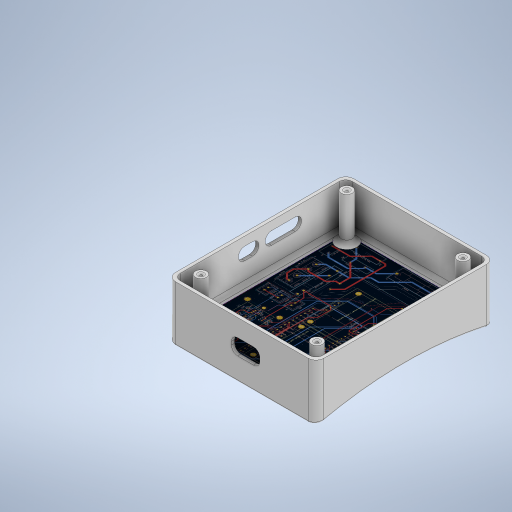
# Autodesk Inventor part: lautering_tank_box
Saved by Autodesk Inventor 2024.4 (Build 284460000, 460)
## iProperties
Created: 2026-05-24
Part Number: lautering_tank_box
Material: Generic
Document SubType Name: Modeling
Designer: Emil
Density: 1 g/cm^3
Appearance: Default
Author: Emil
Autodesk Inventor part; units mm, degrees
ref_plane "YZ Plane" through (0, 0, 0) normal (1, 0, 0) x (0, 1, 0)
ref_plane "XZ Plane" through (0, 0, 0) normal (0, 1, 0) x (-1, 0, 0)
ref_plane "XY Plane" through (0, 0, 0) normal (0, 0, 1) x (1, 0, 0)
sketch "Sketch1" plane through (0, 0, 0) normal (0, 1, 0) x (-1, 0, 0)
  line L0 (0, 0) -> (0, -100.838) construction
  line L1 (0, -100.838) -> (-82.0304, -100.838) construction
  line L2 (-82.0304, -100.838) -> (-82.0304, 0) construction
  line L3 (-82.0304, 0) -> (0, 0) construction
  point P0 (-41.0152, -50.419)
  point P1 (-41.0152, -50.419)
  constraints: 4 other
sketch "Sketch2" plane through (0, 0, 0) normal (0, 1, 0) x (-1, 0, 0)
  line L0 (-86.0304, 4) -> (4, 4)
  line L1 (4, 4) -> (4, -104.838)
  line L2 (4, -104.838) -> (-86.0304, -104.838)
  line L3 (-86.0304, -104.838) -> (-86.0304, 4)
  line L4 (-86.0304, 4) -> (4, -104.838) construction
  line L5 (4, 4) -> (-86.0304, -104.838) construction
  line L6 (-88.0304, 6) -> (6, 6)
  line L7 (6, 6) -> (6, -106.838)
  line L8 (6, -106.838) -> (-88.0304, -106.838)
  line L9 (-88.0304, -106.838) -> (-88.0304, 6)
  line L10 (-88.0304, 6) -> (6, -106.838) construction
  line L11 (6, 6) -> (-88.0304, -106.838) construction
  line L12 (0, -100.838) -> (-82.0304, -100.838) construction
  line L13 (-82.0304, 0) -> (0, 0) construction
  line L14 (0, 0) -> (0, -100.838) construction
  line L15 (-82.0304, -100.838) -> (-82.0304, 0) construction
  point P0 (-41.0152, -50.419)
  dimension "d28" = 4
  dimension "d29" = 2
  dimension "d30" = 4
  dimension "d31" = 2
  dimension "d96" = 94.0304
  dimension "d97" = 112.838
  constraints: 24 end point, 4 midpoint, 4 parallel, 2 horizontal, 2 perpendicular
  measures "d28" distance between parallel lines of L2 L12
  measures "d29" distance between parallel lines of L8 L2
  measures "d30" distance between parallel lines of L1 L14
  measures "d31" distance between parallel lines of L7 L1
  measures "d96" distance of L7.end L8.end
  measures "d97" distance of L8.end L6.start
extrude "Extrusion1" add sketch "Sketch2" along normal blind 26.5
sketch "Sketch3" plane through (0, 0, 0) normal (0, -1, 0) x (1, 0, 0)
  line L0 (-6, -106.838) -> (-6, 6) projected
  line L1 (88.0304, -106.838) -> (-6, -106.838) projected
  line L2 (-6, 6) -> (88.0304, 6)
  line L3 (88.0304, 6) -> (88.0304, -106.838)
  line L4 (88.0304, -106.838) -> (-6, -106.838)
  line L5 (-6, -106.838) -> (-6, 6)
  point P0 (0, 0)
  constraints: 8 end point, 2 parallel, 1 horizontal, 1 perpendicular
extrude "Extrusion2" add sketch "Sketch3" along normal blind 2
sketch "Sketch4" plane through (0, 0, 0) normal (0, 1, 0) x (1, 0, 0)
  circle A0 centre (4.568, 4.6101) radius 3.5
  circle A1 centre (4.568, 96.895) radius 3.5
  circle A2 centre (78.0955, 96.895) radius 3.5
  circle A3 centre (77.9805, 4.6404) radius 3.5
  point P0 (0, 0)
  dimension "d38" = 7
  dimension "d39" = 7
  dimension "d40" = 7
  dimension "d41" = 7
  constraints: 4 centre point
  measures "d38" diameter of A0
  measures "d39" diameter of A1
  measures "d40" diameter of A2
  measures "d41" diameter of A3
extrude "Extrusion3" add sketch "Sketch4" along normal blind 28
sketch "Sketch5" plane through (4.568, 28, -4.6101) normal (0, 1, 0) x (1, 0, 0)
  circle A0 centre (0, 0) radius 3.5 projected
  circle A1 centre (0, 0) radius 1
  circle A2 centre (0, 92.2849) radius 3.5 projected
  circle A3 centre (73.5275, 92.2849) radius 3.5 projected
  circle A4 centre (73.4125, 0.0303) radius 3.5 projected
  circle A5 centre (73.5275, 92.2849) radius 1
  circle A6 centre (73.4125, 0.0303) radius 1
  circle A7 centre (0, 92.2849) radius 1
  point P0 (-4.568, -4.6101)
  dimension "d45" = 2
  dimension "d46" = 2
  dimension "d47" = 2
  dimension "d48" = 2
  constraints: 4 centre point, 4 coincident
  measures "d45" diameter of A1
  measures "d46" diameter of A5
  measures "d47" diameter of A6
  measures "d48" diameter of A7
extrude "Extrusion4" cut sketch "Sketch5" against normal blind 12 contours A1 | A5 | A6 | A7
fillet "Fillet4" radius 3 4 edges at (1.068, 0, -4.6101) (1.068, 0, -96.895) (74.4805, 0, -4.6404) (74.5955, 0, -96.895)
fillet "Fillet5" radius 2.3 4 edges at (-4, 0, -50.419) (41.0152, 0, -104.838) (41.0152, 0, 4) (86.0304, 0, -50.419)
sketch "Sketch6" plane through (0, -2, 0) normal (0, -1, 0) x (1, 0, 0)
  line L0 (88.0304, 6) -> (-6, 6) projected
  line L1 (88.0304, 6) -> (-6, 6)
  line L2 (-6, 6) -> (-6, -106.838)
  line L3 (-6, -106.838) -> (88.0304, -106.838)
  line L4 (88.0304, -106.838) -> (88.0304, 6)
  arc A0 (-4, -102.538) -> (-1.7, -104.838) centre (-1.7, -102.538) ccw projected
  arc A1 (83.7304, -104.838) -> (86.0304, -102.538) centre (83.7304, -102.538) ccw projected
  arc A2 (86.0304, 1.7) -> (83.7304, 4) centre (83.7304, 1.7) ccw projected
  line L5 (83.0304, 1) -> (-1, 1)
  line L6 (-1, 1) -> (-1, -101.838)
  line L7 (-1, -101.838) -> (83.0304, -101.838)
  line L8 (83.0304, -101.838) -> (83.0304, 1)
  line L9 (-6, -106.838) -> (88.0304, -106.838)
  line L10 (88.0304, -106.838) -> (88.0304, 6)
  line L11 (88.0304, 6) -> (-6, 6)
  line L12 (-6, 6) -> (-6, -106.838)
  point P0 (0, 0)
  point P1 (-6, 6)
  dimension "d62" = 5
  dimension "d63" = 5
  dimension "d64" = 5
  dimension "d65" = 5
  constraints: 24 end point, 6 parallel, 3 horizontal, 3 perpendicular
  measures "d62" distance between parallel lines of L5 L0
  measures "d63" distance between parallel lines of L2 L6
  measures "d64" distance between parallel lines of L3 L7
  measures "d65" distance between parallel lines of L4 L8
extrude "Extrusion5" add sketch "Sketch6" along normal blind 7
sketch "Sketch7" plane through (88.0304, 26.5, 6) normal (1, 0, 0) x (0, 0, -1)
  line L0 (112.838, 0) -> (112.838, -35.5) projected
  line L1 (0, -35.5) -> (0, 0) projected
  arc A0 (112.838, -35.5) -> (0, -35.5) centre (56.419, -268.7743) ccw
  line L2 (0, -35.5) -> (112.838, -35.5)
  point P0 (6, -26.5)
  dimension "d56" = 112.838
  dimension "d57" = 240
  constraints: 2 end point, 2 point on circle, 1 centre point, 1 perpendicular
  measures "d56" distance between parallel lines of L0 L1
  measures "d57" radius of A0
extrude "Extrusion6" cut sketch "Sketch7" against normal up to surface (94.0304 mm away)
fillet "Fillet6" radius 5 4 edges at (88.0304, 8.75, 6) (88.0304, 8.75, -106.838) (-6, 8.75, 6) (-6, 8.75, -106.838)
fillet "Fillet7" radius 4 8 edges at (-1, -4.9236, 1) (83.0304, -4.9236, 1) (83.0304, -4.9236, -101.838) (-1, -4.9236, -101.838) (41.0152, -2, -101.838) (-1, -2, -50.419) (83.0304, -2, -50.419) (41.0152, -2, 1)
fillet "Fillet8" radius 1 4 edges at (77.0955, 28, -96.895) (76.9805, 28, -4.6404) (3.568, 28, -4.6101) (3.568, 28, -96.895)
sketch "Sketch8" plane through (-6, -7.8471, -101.838) normal (-1, 0, 0) x (0, 0, 1)
  line L0 (65, 20.8471) -> (65, 28.8471)
  line L1 (25, 28.8471) -> (25, 20.8471)
  line L2 (25, 20.8471) -> (65, 28.8471) construction
  line L3 (65, 20.8471) -> (25, 28.8471) construction
  line L4 (95.5069, 7.8471) -> (6.6641, 7.8471) projected
  line L5 (0, 0) -> (0, 34.3471) projected
  line L6 (52, 20.8471) -> (52, 28.8471)
  line L7 (48, 28.8471) -> (48, 20.8471)
  line L8 (25, 20.8471) -> (48, 20.8471)
  line L9 (52, 20.8471) -> (65, 20.8471)
  line L10 (65, 28.8471) -> (52, 28.8471)
  line L11 (48, 28.8471) -> (25, 28.8471)
  line L12 (8.443, 35.8471) -> (1.443, 35.8471) projected
  point P0 (101.838, 7.8471)
  point P1 (45, 24.8471)
  point P2 (4.943, 35.8471)
  dimension "d70" = 8
  dimension "d71" = 40
  dimension "d74" = 25
  dimension "d80" = 13
  dimension "d81" = 23
  dimension "d92" = 7
  dimension "d93" = 7
  constraints: 20 end point, 6 parallel, 3 midpoint, 2 horizontal, 2 perpendicular
  measures "d70" distance of L1.start L1.end
  measures "d71" distance of L0.end L1.start
  measures "d74" distance between parallel lines of L5 L1
  measures "d80" distance of L0.end L6.end
  measures "d81" distance of L7.start L1.start
  measures "d92" distance between parallel lines of L12 L11
  measures "d93" distance from line of point (4.943, 35.847) L10
extrude "Extrusion7" cut sketch "Sketch8" against normal up to surface (2 mm away)
fillet "Fillet10" radius 4 8 edges at (-5, 13, -76.838) (-5, 21, -76.838) (-5, 13, -36.838) (-5, 21, -36.838) (-5, 13, -49.838) (-5, 21, -49.838) (-5, 21, -53.838) (-5, 13, -53.838)
fillet "Fillet11" radius 4 8 edges at (-3.3263, 0.6737, 3.3263) (-4, 14.4, 4) (85.3568, 0.6737, 3.3263) (86.0304, 14.4, 4) (85.3568, 0.6737, -104.1643) (86.0304, 14.4, -104.838) (-3.3263, 0.6737, -104.1643) (-4, 14.4, -104.838)
sketch "Sketch9" plane through (-1, -9, 6) normal (0, 0, 1) x (1, 0, 0)
  line L0 (35.5, 24.5) -> (53.5, 24.5)
  line L1 (53.5, 24.5) -> (53.5, 14.5)
  line L2 (53.5, 14.5) -> (35.5, 14.5)
  line L3 (35.5, 14.5) -> (35.5, 24.5)
  line L4 (-5, 35.5) -> (-5, 1.1529) projected
  line L5 (80.0304, 3) -> (4, 3) projected
  line L6 (0, 35.5) -> (84.0304, 35.5) projected
  line L7 (9.068, 37) -> (2.068, 37) projected
  point P0 (1, 9)
  dimension "d85" = 10
  dimension "d86" = 18
  dimension "d87" = 40.5
  dimension "d90" = 12.5
  constraints: 8 end point, 2 parallel, 1 horizontal, 1 perpendicular
  measures "d85" distance of L2.end L0.start
  measures "d86" distance of L0.start L0.end
  measures "d87" distance between parallel lines of L4 L3
  measures "d90" distance between parallel lines of L0 L7
extrude "Extrusion8" cut sketch "Sketch9" against normal up to surface (2 mm away)
fillet "Fillet12" radius 4 4 edges at (34.5, 5.5, 5) (52.5, 15.5, 5) (52.5, 5.5, 5) (34.5, 15.5, 5)
fillet "Fillet13" radius 1 8 edges at (86.3072, -8.7075, -105.6146) (41.0152, -9, -106.838) (-4.2757, -8.7077, -105.6156) (-6, -2.2743, -50.419) (-4.2768, -8.7075, 4.7766) (41.0152, -9, 6) (86.3286, -8.7031, 4.7579) (88.0304, -2.2743, -50.419)
body "Solid1"
